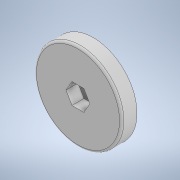
# Autodesk Inventor part: kikcer_head_002
Saved by Autodesk Inventor 2020 (Build 240168000, 168)
## iProperties
Created: 2023-10-29
Part Number: kikcer_head_002
Material: Типовые
Document SubType Name: Modeling
Designer: denis
Density: 1 g/cm^3
Appearance: По умолчанию
Author: denis
Autodesk Inventor part; units mm, degrees
ref_plane "YZ Plane" through (0, 0, 0) normal (1, 0, 0) x (0, 1, 0)
ref_plane "XZ Plane" through (0, 0, 0) normal (0, 1, 0) x (-1, 0, 0)
sketch "Эскиз1" plane through (0, 0, 0) normal (0, 1, 0) x (-1, 0, 0)
  line L0 (-10, 1.75) -> (10, 1.75)
  line L1 (10, 1.75) -> (10, -1.75)
  line L2 (10, -1.75) -> (-10, -1.75)
  line L3 (-10, -1.75) -> (-10, 1.75)
  line L4 (-10, 1.75) -> (10, -1.75) construction
  line L5 (10, 1.75) -> (-10, -1.75) construction
  line L6 (2.5, -1.75) -> (-2.5, -1.75)
  line L7 (-2.5, -1.75) -> (-2.5, -3.75)
  line L8 (-2.5, -3.75) -> (2.5, -3.75)
  line L9 (2.5, -3.75) -> (2.5, -1.75)
  line L10 (0, 1.75) -> (0, -1.75)
  point P0 (0, 0)
  dimension "d0" = 20
  dimension "d1" = 3.5
  dimension "d2" = 5
  dimension "d3" = 2
  constraints: 22 end point, 5 midpoint, 4 parallel, 2 horizontal, 2 perpendicular, 1 vertical
  measures "d0" distance of L1.end L2.end
  measures "d1" distance of L0.end L1.end
  measures "d2" distance of L8.end L7.end
  measures "d3" distance of L7.end L6.end
revolve "Вращение1" add sketch "Эскиз1" angle 360 about axis through (0, 0, 1.75) along (0, 0, -1) contours L0 L1 L2 L10
ref_plane "РабПлоскость2" through (-7.5, 5, 1.5) normal (0, 0, 1) x (1, 0, 0)
sketch "Эскиз3" plane through (-7.5, 5, 1.5) normal (0, 0, 1) x (1, 0, 0)
  circle A0 centre (7.5, -5) radius 2.725 construction
  line L0 (7.5, -5) -> (8.8625, -2.6401) construction
  line L1 (7.5, -5) -> (6.1375, -2.6401) construction
  line L2 (7.5, -5) -> (4.775, -5) construction
  line L3 (7.5, -5) -> (6.1375, -7.3599) construction
  line L4 (7.5, -5) -> (8.8625, -7.3599) construction
  line L5 (7.5, -5) -> (10.225, -5) construction
  line L6 (6.1375, -2.6401) -> (8.8625, -2.6401)
  line L7 (8.8625, -2.6401) -> (10.225, -5)
  line L8 (10.225, -5) -> (8.8625, -7.3599)
  line L9 (6.1375, -7.3599) -> (8.8625, -7.3599)
  line L10 (4.775, -5) -> (6.1375, -7.3599)
  line L11 (4.775, -5) -> (6.1375, -2.6401)
  dimension "d12" = 5.45
  dimension "d15" = 360
  constraints: 24 end point, 3 parallel, 1 coincident, 1 horizontal, 22 other
extrude "Выдавливание4" cut sketch "Эскиз3" along normal blind 2.5 and the other way blind 2.5
sketch "Эскиз4" plane through (0, 0, -1.75) normal (0, 0, -1) x (-1, 0, 0)
  circle A0 centre (0, 0) radius 1.3
  circle A1 centre (0, 0) radius 4.5
  point P0 (0, 0)
  dimension "d20" = 2.6
  dimension "d21" = 9
  constraints: 2 centre point, 2 coincident
  measures "d20" diameter of A0
  measures "d21" diameter of A1
extrude "Выдавливание5" add sketch "Эскиз4" along normal blind 2
extrude "Выдавливание6" cut sketch "Эскиз4" against normal mid plane 12 contours A0
fillet "Сопряжение1" radius 0.5 1 edges at (10, 0, 1.75)
